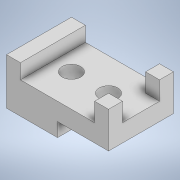
# Autodesk Inventor part: 2.2
Saved by Autodesk Inventor 2022 (Build 260153000, 153)
## iProperties
Created: 2023-04-17
Part Number: 2.2
Material: Genérico
Document SubType Name: Modeling
Designer: jpjoa
Density: 1 g/cm^3
Appearance: Padrão
Author: jpjoa
Autodesk Inventor part; units mm, degrees
ref_plane "YZ Plane" through (0, 0, 0) normal (1, 0, 0) x (0, 1, 0)
ref_plane "XZ Plane" through (0, 0, 0) normal (0, 1, 0) x (-1, 0, 0)
ref_plane "XY Plane" through (0, 0, 0) normal (0, 0, 1) x (1, 0, 0)
sketch "Esboço1" plane through (0, 0, 0) normal (0, 0, 1) x (1, 0, 0)
  line L0 (0, 0) -> (55, 0)
  line L1 (0, 0) -> (0, 50)
  line L2 (0, 50) -> (15, 50)
  line L3 (15, 50) -> (15, 34)
  line L4 (55, 0) -> (55, 15)
  line L5 (55, 15) -> (110, 15)
  line L6 (15, 34) -> (110, 34)
  line L7 (110, 34) -> (110, 15)
  dimension "d0" = 55
  dimension "d1" = 50
  dimension "d2" = 15
  dimension "d3" = 16
  dimension "d7" = 15
  dimension "d8" = 55
  dimension "d9" = 95
  constraints: 16 end point, 3 perpendicular, 2 horizontal, 2 vertical
  measures "d0" distance of L0.start L0.end
  measures "d1" distance of L0.start L1.end
  measures "d2" distance of L1.end L2.end
  measures "d3" distance of L2.end L3.end
  measures "d7" distance of L0.end L4.end
  measures "d8" distance of L4.end L5.end
  measures "d9" distance of L3.end L6.end
extrude "Extrusão1" add sketch "Esboço1" against normal blind 70
sketch "Esboço4" plane through (15, 34, 0) normal (0, 1, 0) x (1, 0, 0)
  circle A0 centre (20, 35) radius 10
  circle A1 centre (60, 35) radius 10
  line L0 (0, 0) -> (0, 70) projected
  line L1 (0, 70) -> (95, 70) projected
  line L2 (95, 0) -> (95, 70) projected
  line L3 (95, 0) -> (80, 0)
  line L4 (80, 0) -> (80, 15)
  line L5 (80, 15) -> (95, 15)
  line L6 (95, 15) -> (95, 0)
  line L7 (95, 70) -> (80, 70)
  line L8 (80, 70) -> (80, 55)
  line L9 (80, 55) -> (95, 55)
  line L10 (95, 55) -> (95, 70)
  point P0 (-15, 0)
  dimension "d19" = 20
  dimension "d20" = 20
  dimension "d21" = 20
  dimension "d22" = 40
  dimension "d23" = 35
  dimension "d24" = 15
  dimension "d25" = 15
  dimension "d26" = 15
  dimension "d27" = 15
  constraints: 16 end point, 4 parallel, 2 centre point, 2 horizontal, 2 perpendicular, 1 horizontal alignment
  measures "d19" diameter of A0
  measures "d20" diameter of A1
  measures "d21" distance from line of L0 A0.centre
  measures "d22" distance of A1.centre A0.centre
  measures "d23" distance from line of L1 A1.centre
  measures "d24" distance of L4.end L5.end
  measures "d25" distance of L3.end L4.end
  measures "d26" distance of L9.end L8.end
  measures "d27" distance of L8.end L7.end
extrude "Extrusão3" cut sketch "Esboço4" against normal through all contours A0 | A1
extrude "Extrusão4" add sketch "Esboço4" along normal blind 20 contours L1 L2 L9 L8 | L3 L4 L5 L2
